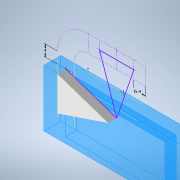
# Autodesk Inventor part: Part7
Saved by Autodesk Inventor 2022 (Build 260153000, 153)
## iProperties
Created: 2024-04-11
Part Number: Part7
Material: Generic
Document SubType Name: Modeling
Designer: Gotham City
Density: 1 g/cm^3
Appearance: Default
Author: Gotham City
Autodesk Inventor part; units mm, degrees
ref_plane "YZ Plane" through (0, 0, 0) normal (1, 0, 0) x (0, 1, 0)
ref_plane "XZ Plane" through (0, 0, 0) normal (0, 1, 0) x (-1, 0, 0)
ref_plane "XY Plane" through (0, 0, 0) normal (0, 0, 1) x (1, 0, 0)
sketch "Sketch1" plane through (0, 0, 0) normal (0, 0, 1) x (1, 0, 0)
  line L0 (-3, 10) -> (-3, -10) construction
  line L1 (3, -10) -> (3, 10) construction
  arc A0 (7.6994, 20.6994) -> (-3, 10) centre (7.6994, 10) ccw construction
  arc A1 (7.6994, 14.6994) -> (3, 10) centre (7.6994, 10) ccw construction
  line L2 (7.6994, 14.6994) -> (7.6994, 20.6994) construction
  line L3 (3, 10) -> (-3, 10) construction
  line L4 (7.6994, 14.6994) -> (27.6994, 14.6994) construction
  line L5 (27.6994, 14.6994) -> (27.6994, 20.6994) construction
  line L6 (27.6994, 20.6994) -> (7.6994, 20.6994) construction
  line L7 (18.62, 8.826) -> (21.52, 8.826) construction
  line L8 (7.27, 2.85) -> (25.1046, 2.85) construction
  line L9 (7.27, 8.826) -> (26.9771, 8.826) construction
  line L10 (3, 6) -> (-3, 6) construction
  line L11 (-3, -6) -> (3, -6) construction
  line L12 (0, 0) -> (-3, 0)
  line L13 (23.6994, 14.6994) -> (23.6994, 20.6994) construction
  line L14 (17.6994, 20.6994) -> (17.6994, 14.6994) construction
  line L15 (11.6994, 14.6994) -> (11.6994, 20.6994) construction
  line L16 (0, 6) -> (0, -6)
  line L17 (0, -6) -> (17.6994, 0)
  line L18 (17.6994, 0) -> (0, 6)
  line L19 (23.6994, 17.6994) -> (17.6994, 0)
  line L20 (11.6994, 17.6994) -> (17.6994, 0)
  line L21 (23.6994, 17.6994) -> (11.6994, 17.6994)
  point P0 (20.07, 8.826)
  dimension "d5" = 4
  dimension "d6" = 4
  constraints: 32 end point, 8 midpoint, 8 point on line, 6 perpendicular, 5 equal length, 4 point on circle, 2 centre point, 2 horizontal, 2 tangent, 1 coincident, 1 vertical, 2 other
  measures "d5" distance between parallel lines of L3 L10
  measures "d6" distance between parallel lines of L5 L13
sketch "Sketch2" plane through (0, 0, 0) normal (0, 0, 1) x (1, 0, 0)
  line L0 (17.6994, 0) -> (0, 6) projected
  line L1 (0, -6) -> (17.6994, 0) projected
  line L2 (0, 6) -> (0, -6) projected
extrude "Extrusion1" add sketch "Sketch2" along normal blind 3
equation "\"d6\" = d5"
body "Solid1"
